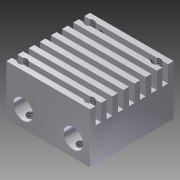
# Autodesk Inventor part: ChimeraHeatsink
Saved by Autodesk Inventor 2015 SP1 (Build 190203100, 203)
## iProperties
Created: 2014-11-28
Part Number: ChimeraHeatsink
Material: Aluminum 6061
Document SubType Name: Modeling
Designer: Jack
Density: 2.7 g/cm^3
Appearance: Aluminum - Flat
Mass: 31.3389 g
Surface Area: 76.0365 cm^2
Volume: 11.607 cm^3
Author: Jack
Autodesk Inventor part; units mm, degrees
ref_plane "YZ Plane" through (0, 0, 0) normal (1, 0, 0) x (0, 1, 0)
ref_plane "XZ Plane" through (0, 0, 0) normal (0, 1, 0) x (-1, 0, 0)
ref_plane "XY Plane" through (0, 0, 0) normal (0, 0, 1) x (1, 0, 0)
sketch "Sketch1" plane through (0, 0, 0) normal (0, 0, 1) x (1, 0, 0)
  line L0 (0, 0) -> (30, 0)
  line L1 (30, 0) -> (30, 30)
  line L2 (30, 30) -> (0, 30)
  line L3 (0, 30) -> (0, 0)
  dimension "d0" = 30
  dimension "d1" = 30
  constraints: 8 end point, 2 parallel, 1 horizontal, 1 perpendicular
  measures "d0" distance of L2.end L1.end
  measures "d1" distance of L1.end L0.end
extrude "Extrusion1" add sketch "Sketch1" along normal blind 12
sketch "Sketch2" plane through (0, 0, 12) normal (0, 0, 1) x (1, 0, 0)
  line L0 (30, 0) -> (30, 30) projected
  line L1 (30, 30) -> (0, 30) projected
  line L2 (0, 30) -> (0, 0) projected
  line L3 (0, 28) -> (30, 28)
  dimension "d7" = 2
  constraints: 2 end point, 2 point on line, 1 horizontal
  measures "d7" distance between parallel lines of L1 L3
extrude "Extrusion2" add sketch "Sketch2" along normal blind 6
pattern_linear "Rectangular Pattern1" count 8 spacing 4 along (0, -1, 0) of "Extrusion2"
sketch "Sketch3" plane through (0, 0, 0) normal (0, -1, 0) x (1, 0, 0)
  line L0 (0, 0) -> (30, 0) projected
  line L1 (0, 0) -> (0, 18) projected
  circle A0 centre (6, 6) radius 3.5
  circle A1 centre (24, 6) radius 3.5
  dimension "d11" = 18
  dimension "d12" = 7
  dimension "d13" = 6
  dimension "d14" = 6
  constraints: 2 centre point, 1 equal radius, 1 horizontal alignment
  measures "d11" distance of A1.centre A0.centre
  measures "d12" diameter of A1
  measures "d13" distance from line of L0 A1.centre
  measures "d14" distance from line of L1 A0.centre
extrude "Extrusion3" cut sketch "Sketch3" against normal blind 15
sketch "Sketch4" plane through (24, 15, 6) normal (0, -1, 0) x (1, 0, 0)
  circle A0 centre (0, 0) radius 3.5 projected
  circle A1 centre (-18, 0) radius 3.5 projected
  circle A2 centre (-18, 0) radius 0.925
  circle A3 centre (0, 0) radius 0.925
  point P0 (-24, -6)
  dimension "d17" = 1.85
  dimension "d18" = 1.85
  constraints: 2 centre point, 2 coincident
  measures "d17" diameter of A2
  measures "d18" diameter of A3
extrude "Extrusion4" cut sketch "Sketch4" against normal up to next contours A2 | A3
sketch "Sketch5" plane through (0, 30, 0) normal (0, 1, 0) x (1, 0, 0)
  circle A0 centre (24, -6) radius 0.925 projected
  circle A1 centre (6, -6) radius 0.925 projected
  line L0 (30, -18) -> (0, -18) projected
  circle A2 centre (24, -15) radius 1.5
  circle A3 centre (6, -15) radius 1.5
  dimension "d21" = 3
  dimension "d22" = 3
  constraints: 2 centre point, 2 vertical alignment, 1 equal radius, 1 horizontal alignment
  measures "d21" diameter of A2
  measures "d22" distance from line of L0 A2.centre
extrude "Extrusion5" cut sketch "Sketch5" against normal up to surface (2 mm away) contours A2 | A3
thread "Thread1" size "M3x0.5" class "6H" standard "ANSI Metric M Profile" full length
thread "Thread2" size "M3x0.5" class "6H" standard "ANSI Metric M Profile" full length
sketch "Sketch6" plane through (0, 0, 18) normal (0, 0, 1) x (1, 0, 0)
  line L0 (30, 28) -> (30, 30)
  line L1 (30, 26) -> (0, 26)
  line L2 (0, 26) -> (0, 24)
  line L3 (0, 24) -> (30, 24)
  line L4 (30, 24) -> (30, 26)
  line L5 (30, 22) -> (0, 22)
  line L6 (0, 22) -> (0, 20)
  line L7 (0, 20) -> (30, 20)
  line L8 (30, 20) -> (30, 22)
  line L9 (30, 18) -> (0, 18)
  line L10 (0, 18) -> (0, 16)
  line L11 (0, 16) -> (30, 16)
  line L12 (30, 16) -> (30, 18)
  line L13 (30, 14) -> (0, 14)
  line L14 (0, 14) -> (0, 12)
  line L15 (0, 12) -> (30, 12)
  line L16 (30, 12) -> (30, 14)
  line L17 (30, 10) -> (0, 10)
  line L18 (0, 10) -> (0, 8)
  line L19 (0, 8) -> (30, 8)
  line L20 (30, 8) -> (30, 10)
  line L21 (30, 6) -> (0, 6)
  line L22 (0, 6) -> (0, 4)
  line L23 (0, 4) -> (30, 4)
  line L24 (30, 4) -> (30, 6)
  line L25 (30, 2) -> (0, 2)
  line L26 (0, 2) -> (0, 0)
  line L27 (0, 0) -> (30, 0)
  line L28 (30, 0) -> (30, 2)
  circle A0 centre (3, 26.8635) radius 1.5
  circle A1 centre (27, 26.8635) radius 1.5
  circle A2 centre (27, 2.8635) radius 1.5
  circle A3 centre (3, 2.8635) radius 1.5
  point P0 (0, 0)
extrude "Extrusion6" cut sketch "Sketch6" against normal up to surface (6 mm away) contours A1 L1 | L1 A1 | A0 L1 | L1 A0 | A2 L25 L23 | L23 A2 | A3 L23 | L23 A3 L25 | L25 A3 | L25 A2
thread "Thread3" size "M3x0.5" class "6H" standard "ANSI Metric M Profile" full length
thread "Thread4" size "M3x0.5" class "6H" standard "ANSI Metric M Profile" full length
thread "Thread5" size "M3x0.5" class "6H" standard "ANSI Metric M Profile" full length
thread "Thread6" size "M3x0.5" class "6H" standard "ANSI Metric M Profile" full length
thread "Thread7" size "M3x0.5" class "6H" standard "ANSI Metric M Profile" full length
thread "Thread8" size "M3x0.5" class "6H" standard "ANSI Metric M Profile" full length
thread "Thread9" size "M3x0.5" class "6H" standard "ANSI Metric M Profile" full length
thread "Thread10" size "M3x0.5" class "6H" standard "ANSI Metric M Profile" full length
sketch "Sketch7" plane through (0, 30, 0) normal (0, 1, 0) x (1, 0, 0)
  circle A0 centre (24, -6) radius 0.925 projected
  circle A1 centre (6, -6) radius 0.925 projected
  circle A2 centre (24, -6) radius 0.925 projected
  circle A3 centre (24, -6) radius 4
  circle A4 centre (6, -6) radius 4
  dimension "d52" = 8
  constraints: 2 centre point, 2 coincident, 1 equal radius
  measures "d52" diameter of A3
extrude "Extrusion7" cut sketch "Sketch7" against normal blind 6
sketch "Sketch8" plane through (0, 0, 0) normal (0, 0, -1) x (-1, 0, 0)
  line L0 (0, 0) -> (-30, 0) projected
  circle A0 centre (-24, 3) radius 1.5
  circle A1 centre (-24, 11) radius 1.5
  circle A2 centre (-6, 11) radius 1.5
  circle A3 centre (-6, 3) radius 1.5
  line L1 (-20.5, 15) -> (-27.5, 15) projected
  line L2 (-20.5, 0) -> (-27.5, 0) projected
  line L3 (-2.5, 15) -> (-9.5, 15) projected
  line L4 (-2.5, 0) -> (-9.5, 0) projected
  dimension "d55" = 3
  dimension "d56" = 8
  dimension "d57" = 3.5
  dimension "d58" = 3.5
  dimension "d59" = 3
  constraints: 4 centre point, 3 equal radius, 2 horizontal alignment, 2 vertical alignment
  measures "d55" diameter of A1
  measures "d56" distance of A2.centre A3.centre
  measures "d57" horizontal distance of L3.end A2.centre
  measures "d58" horizontal distance of L1.start A1.centre
  measures "d59" distance from line of L0 A0.centre
extrude "Extrusion8" cut sketch "Sketch8" against normal up to next
thread "Thread11" size "M3x0.5" class "6H" standard "ANSI Metric M Profile" full length
thread "Thread12" size "M3x0.5" class "6H" standard "ANSI Metric M Profile" full length
thread "Thread13" size "M3x0.5" class "6H" standard "ANSI Metric M Profile" full length
thread "Thread14" size "M3x0.5" class "6H" standard "ANSI Metric M Profile" full length
sketch "Sketch9" plane through (0, 0, 0) normal (0, 0, -1) x (-1, 0, 0)
  line L0 (-30, 0) -> (-30, 30) projected
  circle A0 centre (-15, 10) radius 1.5
  circle A1 centre (-19.5, 20) radius 1.5
  circle A2 centre (-10.5, 20) radius 1.5
  line L1 (0, 22) -> (-30, 22) projected
  line L2 (0, 0) -> (-30, 0) projected
  dimension "d70" = 3
  dimension "d73" = 10.5
  dimension "d75" = 10
  dimension "d84" = 19.5
  dimension "d85" = 15
  dimension "d86" = 20
  constraints: 3 centre point, 2 equal radius, 1 horizontal alignment
  measures "d70" diameter of A0
  measures "d73" distance from line of L0 A1.centre
  measures "d75" vertical distance of A1.centre A0.centre
  measures "d84" distance from line of L0 A2.centre
  measures "d85" distance from line of L0 A0.centre
  measures "d86" distance from line of L2 A2.centre
extrude "Extrusion9" cut sketch "Sketch9" against normal blind 6
thread "Thread15" size "M3x0.5" class "6H" standard "ANSI Metric M Profile" full length
thread "Thread16" size "M3x0.5" class "6H" standard "ANSI Metric M Profile" full length
thread "Thread17" size "M3x0.5" class "6H" standard "ANSI Metric M Profile" full length
body "Solid1"
